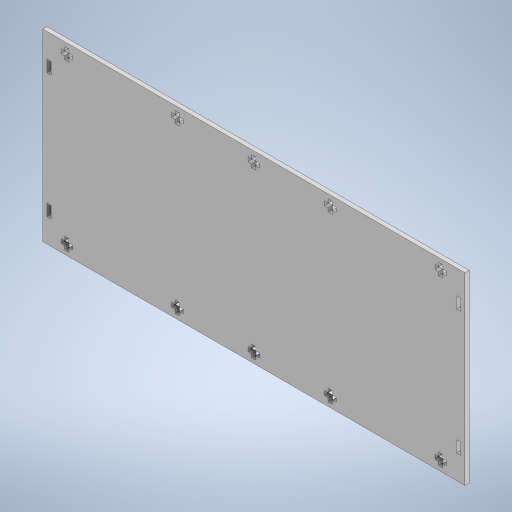
# Autodesk Inventor part: plate_expansion
Saved by Autodesk Inventor 2023 (Build 270158000, 158)
## iProperties
Created: 2023-05-04
Part Number: plate_expansion
Material: 一般
Document SubType Name: Modeling
Designer: 陳詩穎
Density: 1 g/cm^3
Appearance: 預設
Author: 陳詩穎
Autodesk Inventor part; units mm, degrees
ref_plane "YZ Plane" through (0, 0, 0) normal (1, 0, 0) x (0, 1, 0)
ref_plane "XZ Plane" through (0, 0, 0) normal (0, 1, 0) x (-1, 0, 0)
ref_plane "XY Plane" through (0, 0, 0) normal (0, 0, 1) x (1, 0, 0)
sketch "草圖1" plane through (0, 0, 0) normal (0, 0, 1) x (1, 0, 0)
  line L0 (-149, 65) -> (149, 65)
  line L1 (149, 65) -> (149, -65)
  line L2 (149, -65) -> (-149, -65)
  line L3 (-149, -65) -> (-149, 65)
  line L4 (0, -91) -> (0, 91) projected
  line L5 (-208.6, 0) -> (208.6, 0) projected
  point P0 (0, 0)
  dimension "d0" = 298
  dimension "d1" = 130
  constraints: 8 end point, 2 parallel, 1 horizontal, 1 perpendicular, 2 other
  measures "d0" distance of L0.start L0.end
  measures "d1" distance of L0.end L1.end
extrude "擠出1" add sketch "草圖1" along normal blind 3
sketch "草圖2" plane through (0, 0, 3) normal (0, 0, 1) x (1, 0, 0)
  line L0 (-1.45, 62) -> (1.45, 62)
  line L1 (1.45, 62) -> (1.45, 54)
  line L2 (1.45, 54) -> (-1.45, 54)
  line L3 (-1.45, 54) -> (-1.45, 62)
  line L4 (-4, 59.45) -> (4, 59.45)
  line L5 (4, 59.45) -> (4, 56.55)
  line L6 (4, 56.55) -> (-4, 56.55)
  line L7 (-4, 56.55) -> (-4, 59.45)
  line L8 (149, 65) -> (-149, 65) projected
  line L9 (1.45, 62) -> (-1.45, 54)
  line L10 (-1.45, 62) -> (1.45, 54)
  line L11 (4, 59.45) -> (-4, 56.55)
  line L12 (-4, 59.45) -> (4, 56.55)
  line L13 (-55.43, 62) -> (-52.53, 62)
  line L14 (-52.53, 62) -> (-52.53, 54)
  line L15 (-52.53, 54) -> (-55.43, 54)
  line L16 (-55.43, 54) -> (-55.43, 62)
  line L17 (-57.98, 59.45) -> (-49.98, 59.45)
  line L18 (-49.98, 59.45) -> (-49.98, 56.55)
  line L19 (-49.98, 56.55) -> (-57.98, 56.55)
  line L20 (-57.98, 56.55) -> (-57.98, 59.45)
  line L21 (-52.53, 62) -> (-55.43, 54)
  line L22 (-55.43, 62) -> (-52.53, 54)
  line L23 (-49.98, 59.45) -> (-57.98, 56.55)
  line L24 (-57.98, 59.45) -> (-49.98, 56.55)
  line L25 (-133.41, 62) -> (-130.51, 62)
  line L26 (-130.51, 62) -> (-130.51, 54)
  line L27 (-130.51, 54) -> (-133.41, 54)
  line L28 (-133.41, 54) -> (-133.41, 62)
  line L29 (-135.96, 56.55) -> (-135.96, 59.45)
  line L30 (-130.51, 62) -> (-133.41, 54)
  line L31 (-133.41, 62) -> (-130.51, 54)
  line L32 (-135.96, 59.45) -> (-127.96, 59.45)
  line L33 (-127.96, 56.55) -> (-135.96, 56.55)
  line L34 (-127.96, 59.45) -> (-135.96, 56.55)
  line L35 (-135.96, 59.45) -> (-127.96, 56.55)
  line L36 (-127.96, 59.45) -> (-127.96, 56.55)
  line L37 (-149, 65) -> (-149, -65) projected
  line L38 (-149, 0) -> (145, 0)
  line L39 (0, 65) -> (0, -65)
  line L40 (55.43, 62) -> (52.53, 62)
  line L41 (52.53, 62) -> (52.53, 54)
  line L42 (52.53, 54) -> (55.43, 54)
  line L43 (55.43, 54) -> (55.43, 62)
  line L44 (57.98, 56.55) -> (57.98, 59.45)
  line L45 (52.53, 62) -> (55.43, 54)
  line L46 (55.43, 62) -> (52.53, 54)
  line L47 (57.98, 59.45) -> (49.98, 59.45)
  line L48 (49.98, 56.55) -> (57.98, 56.55)
  line L49 (49.98, 59.45) -> (57.98, 56.55)
  line L50 (57.98, 59.45) -> (49.98, 56.55)
  line L51 (49.98, 59.45) -> (49.98, 56.55)
  line L52 (127.96, 59.45) -> (127.96, 56.55)
  line L53 (130.51, 62) -> (130.51, 54)
  line L54 (133.41, 54) -> (133.41, 62)
  line L55 (130.51, 62) -> (133.41, 54)
  line L56 (133.41, 62) -> (130.51, 54)
  line L57 (130.51, 54) -> (133.41, 54)
  line L58 (135.96, 59.45) -> (127.96, 59.45)
  line L59 (135.96, 59.45) -> (127.96, 56.55)
  line L60 (135.96, 56.55) -> (135.96, 59.45)
  line L61 (127.96, 56.55) -> (135.96, 56.55)
  line L62 (127.96, 59.45) -> (135.96, 56.55)
  line L63 (133.41, 62) -> (130.51, 62)
  line L64 (-1.45, -62) -> (1.45, -62)
  line L65 (1.45, -62) -> (1.45, -54)
  line L66 (1.45, -54) -> (-1.45, -54)
  line L67 (-1.45, -54) -> (-1.45, -62)
  line L68 (-4, -59.45) -> (4, -59.45)
  line L69 (4, -59.45) -> (4, -56.55)
  line L70 (4, -56.55) -> (-4, -56.55)
  line L71 (-4, -56.55) -> (-4, -59.45)
  line L72 (1.45, -62) -> (-1.45, -54)
  line L73 (-1.45, -62) -> (1.45, -54)
  line L74 (4, -59.45) -> (-4, -56.55)
  line L75 (-4, -59.45) -> (4, -56.55)
  line L76 (-55.43, -62) -> (-52.53, -62)
  line L77 (-52.53, -62) -> (-52.53, -54)
  line L78 (-52.53, -54) -> (-55.43, -54)
  line L79 (-55.43, -54) -> (-55.43, -62)
  line L80 (-57.98, -56.55) -> (-57.98, -59.45)
  line L81 (-52.53, -62) -> (-55.43, -54)
  line L82 (-55.43, -62) -> (-52.53, -54)
  line L83 (-57.98, -59.45) -> (-49.98, -59.45)
  line L84 (-49.98, -56.55) -> (-57.98, -56.55)
  line L85 (-49.98, -59.45) -> (-57.98, -56.55)
  line L86 (-57.98, -59.45) -> (-49.98, -56.55)
  line L87 (-49.98, -59.45) -> (-49.98, -56.55)
  line L88 (-127.96, -59.45) -> (-127.96, -56.55)
  line L89 (-130.51, -62) -> (-130.51, -54)
  line L90 (-133.41, -54) -> (-133.41, -62)
  line L91 (-130.51, -62) -> (-133.41, -54)
  line L92 (-133.41, -62) -> (-130.51, -54)
  line L93 (-130.51, -54) -> (-133.41, -54)
  line L94 (-135.96, -59.45) -> (-127.96, -59.45)
  line L95 (-135.96, -59.45) -> (-127.96, -56.55)
  line L96 (-135.96, -56.55) -> (-135.96, -59.45)
  line L97 (-127.96, -56.55) -> (-135.96, -56.55)
  line L98 (-127.96, -59.45) -> (-135.96, -56.55)
  line L99 (-133.41, -62) -> (-130.51, -62)
  line L100 (52.53, -62) -> (52.53, -54)
  line L101 (52.53, -62) -> (55.43, -54)
  line L102 (55.43, -62) -> (52.53, -54)
  line L103 (55.43, -62) -> (52.53, -62)
  line L104 (57.98, -56.55) -> (57.98, -59.45)
  line L105 (57.98, -59.45) -> (49.98, -59.45)
  line L106 (49.98, -56.55) -> (57.98, -56.55)
  line L107 (49.98, -59.45) -> (57.98, -56.55)
  line L108 (55.43, -54) -> (55.43, -62)
  line L109 (52.53, -54) -> (55.43, -54)
  line L110 (49.98, -59.45) -> (49.98, -56.55)
  line L111 (57.98, -59.45) -> (49.98, -56.55)
  line L112 (127.96, -59.45) -> (127.96, -56.55)
  line L113 (130.51, -54) -> (133.41, -54)
  line L114 (130.51, -62) -> (130.51, -54)
  line L115 (133.41, -62) -> (130.51, -62)
  line L116 (133.41, -54) -> (133.41, -62)
  line L117 (133.41, -62) -> (130.51, -54)
  line L118 (130.51, -62) -> (133.41, -54)
  line L119 (127.96, -56.55) -> (135.96, -56.55)
  line L120 (135.96, -59.45) -> (127.96, -59.45)
  line L121 (135.96, -59.45) -> (127.96, -56.55)
  line L122 (127.96, -59.45) -> (135.96, -56.55)
  line L123 (135.96, -56.55) -> (135.96, -59.45)
  line L124 (-146, 48) -> (-143.1, 48)
  line L125 (-143.1, 48) -> (-143.1, 40)
  line L126 (-143.1, 40) -> (-146, 40)
  line L127 (-146, 40) -> (-146, 48)
  line L128 (-146, -40) -> (-143.1, -40)
  line L129 (-143.1, -40) -> (-143.1, -48)
  line L130 (-143.1, -48) -> (-146, -48)
  line L131 (-146, -48) -> (-146, -40)
  line L132 (146, 48) -> (143.1, 48)
  line L133 (143.1, 48) -> (143.1, 40)
  line L134 (143.1, 40) -> (146, 40)
  line L135 (146, 40) -> (146, 48)
  line L136 (146, -40) -> (143.1, -40)
  line L137 (143.1, -40) -> (143.1, -48)
  line L138 (143.1, -48) -> (146, -48)
  line L139 (146, -48) -> (146, -40)
  point P0 (0, 0)
  point P1 (0, 58)
  point P2 (0, 58)
  point P3 (-53.98, 58)
  point P4 (-53.98, 58)
  point P5 (-53.98, 58)
  point P6 (0, 58)
  point P7 (-131.96, 58)
  point P8 (-131.96, 58)
  point P9 (-131.96, 58)
  point P10 (53.98, 58)
  point P11 (53.98, 58)
  point P12 (53.98, 58)
  point P13 (131.96, 58)
  point P14 (131.96, 58)
  point P15 (131.96, 58)
  point P16 (0, -58)
  point P17 (0, -58)
  point P18 (-53.98, -58)
  point P19 (-53.98, -58)
  point P20 (-53.98, -58)
  point P21 (0, -58)
  point P22 (-131.96, -58)
  point P23 (-131.96, -58)
  point P24 (-131.96, -58)
  point P25 (53.98, -58)
  point P26 (53.98, -58)
  point P27 (53.98, -58)
  point P28 (131.96, -58)
  point P29 (131.96, -58)
  point P30 (131.96, -58)
  point P31 (-133.41, -59.45)
  point P32 (-130.51, -59.45)
  point P33 (-130.51, -56.55)
  point P34 (-133.41, -56.55)
  point P35 (-55.43, -56.55)
  point P36 (-55.43, -59.45)
  point P37 (-52.53, -59.45)
  point P38 (-52.53, -56.55)
  point P39 (1.45, -56.55)
  point P40 (-1.45, -56.55)
  point P41 (-1.45, -59.45)
  point P42 (1.45, -59.45)
  point P43 (55.43, -59.45)
  point P44 (55.43, -56.55)
  point P45 (52.53, -56.55)
  point P46 (52.53, -59.45)
  point P47 (133.41, -56.55)
  point P48 (130.51, -56.55)
  point P49 (130.51, -59.45)
  point P50 (133.41, -59.45)
  point P51 (133.41, 59.45)
  point P52 (130.51, 59.45)
  point P53 (130.51, 56.55)
  point P54 (133.41, 56.55)
  point P55 (52.53, 56.55)
  point P56 (55.43, 56.55)
  point P57 (55.43, 59.45)
  point P58 (52.53, 59.45)
  point P59 (-1.45, 59.45)
  point P60 (-1.45, 56.55)
  point P61 (1.45, 56.55)
  point P62 (1.45, 59.45)
  point P63 (-52.53, 59.45)
  point P64 (-55.43, 59.45)
  point P65 (-55.43, 56.55)
  point P66 (-52.53, 56.55)
  point P67 (-130.51, 59.45)
  point P68 (-133.41, 59.45)
  point P69 (-133.41, 56.55)
  point P70 (-130.51, 56.55)
  dimension "d4" = 2.9
  dimension "d5" = 8
  dimension "d6" = 3
  dimension "d7" = 2.9
  dimension "d8" = 8
  dimension "d9" = 51.08
  dimension "d10" = 2.9
  dimension "d11" = 8
  dimension "d13" = 75.08
  dimension "d16" = 2.9
  dimension "d17" = 8
  dimension "d18" = 3
  dimension "d19" = 80
  constraints: 276 end point, 85 symmetric about line, 16 parallel, 14 midpoint, 14 perpendicular, 9 horizontal, 4 point on line, 2 horizontal alignment, 1 vertical, 1 vertical alignment, 2 other
  measures "d4" distance of L0.start L0.end
  measures "d5" distance of L0.end L1.end
  measures "d6" distance from line of L39.start L0
  measures "d7" distance of L13.start L13.end
  measures "d8" distance of L13.end L14.end
  measures "d9" distance between parallel lines of L14 L3
  measures "d10" distance of L28.end L26.start
  measures "d11" distance of L26.start L26.end
  measures "d13" distance between parallel lines of L26 L16
  measures "d16" distance of L124.start L124.end
  measures "d17" distance of L124.end L125.end
  measures "d18" distance between parallel lines of L37 L127
  measures "d19" distance between parallel lines of L128 L126
extrude "擠出2" cut sketch "草圖2" against normal blind 3 contours L10 L4 L3 | L0 L39 L4 L10 | L0 L9 L4 L39 | L4 L10 L12 L3 | L3 L12 L4 | L4 L39 L10 | L1 L4 L9 | L4 L9 L39 | L12 L11 L3 | L3 L11 L7 L12 | L39 L6 L9 | L12 L1 L6 L10 | L9 L4 L1 L11 | L9 L6 L3 L11 | L11 L1 L12 | L10 L6 L39 | L4 L11 L1 | L3 L6 L11 | L9 L3 L6 | L6 L39 L2 L9 | L10 L2 L39 L6 | L6 L1 L10 | L11 L5 L12 L1 | L12 L6 L1 | L22 L17 L16 | L13 L21 L17 L22 | L14 L17 L21 | L17 L22 L24 L16 | L16 L24 L17 | L17 L21 L22 | L17 L23 L14 | L14 L23 L21 L17 | L24 L23 L16 | L16 L23 L20 L24 | L22 L19 L21 | L24 L14 L19 L22 | L21 L19 L16 L23 | L23 L14 L24 | L23 L18 L24 L14 | L16 L19 L23 | L21 L16 L19 | L19 L22 L15 L21 | L19 L14 L22 | L24 L19 L14 | L31 L32 L28 | L25 L30 L32 L31 | L26 L32 L30 | L32 L31 L35 L28 | L28 L35 L32 | L32 L30 L31 | L32 L34 L26 | L26 L34 L30 L32 | L35 L34 L28 | L28 L34 L29 L35 | L31 L33 L30 | L35 L26 L33 L31 | L30 L33 L28 L34 | L34 L26 L35 | L34 L36 L35 L26 | L28 L33 L34 | L33 L31 L27 L30 | L30 L28 L33 | L33 L26 L31 | L35 L33 L26 | L66 L73 L70 L39 | L39 L70 L72 L66 | L70 L73 L39 | L39 L72 L70 | L65 L70 L73 | L72 L70 L67 | L72 L68 L39 | L74 L65 L68 L72 | L74 L67 L70 L72 | L39 L68 L73 | L75 L65 L74 | L75 L67 L74 | L73 L68 L67 L75 | L73 L70 L65 L75 | L70 L75 L65 | L67 L74 L70 | L68 L72 L64 L39 | L39 L64 L73 L68 | L68 L65 L72 | L73 L67 L68 | L74 L68 L65 | L65 L75 L69 L74 | L67 L75 L71 L74 | L67 L68 L75 | L46 L47 L45 L40 | L43 L47 L46 | L45 L47 L41 | L47 L50 L43 | L43 L50 L46 L47 | L46 L45 L47 | L47 L45 L49 L41 | L41 L49 L47 | L50 L44 L49 L43 | L43 L49 L50 | L49 L43 L48 L45 | L45 L48 L46 | L50 L41 L49 | L46 L48 L41 L50 | L41 L50 L51 L49 | L49 L48 L43 | L48 L43 L45 | L45 L42 L46 L48 | L46 L41 L48 | L41 L48 L50 | L62 L53 L59 L52 | L58 L53 L62 | L59 L53 L61 | L58 L55 L62 L53 | L53 L55 L58 | L62 L59 L53 | L59 L56 L61 L53 | L61 L56 L53 | L63 L56 L58 L55 | L58 L56 L55 | L62 L54 L61 L55 | L55 L61 L56 | L56 L58 L54 L59 | L59 L54 L62 | L56 L61 L55 L57 | L54 L58 L56 | L61 L54 L55 | L59 L60 L62 L54 | L54 L58 L59 | L62 L61 L54 | L82 L83 L81 L76 | L79 L83 L82 | L81 L83 L77 | L83 L86 L79 | L79 L86 L82 L83 | L82 L81 L83 | L83 L81 L85 L77 | L77 L85 L83 | L86 L80 L85 L79 | L79 L85 L86 | L85 L79 L84 L81 | L81 L84 L82 | L86 L77 L85 | L82 L84 L77 L86 | L77 L86 L87 L85 | L85 L84 L79 | L84 L79 L81 | L81 L78 L82 L84 | L82 L77 L84 | L77 L84 L86 | L98 L89 L95 L88 | L94 L89 L98 | L95 L89 L97 | L94 L91 L98 L89 | L89 L91 L94 | L98 L95 L89 | L95 L92 L97 L89 | L97 L92 L89 | L99 L92 L94 L91 | L94 L92 L91 | L98 L90 L97 L91 | L91 L97 L92 | L92 L94 L90 L95 | L95 L90 L98 | L92 L97 L91 L93 | L90 L94 L92 | L97 L90 L91 | L95 L96 L98 L90 | L90 L94 L95 | L98 L97 L90 | L100 L105 L101 | L101 L105 L102 L103 | L105 L107 L100 | L100 L107 L101 L105 | L101 L102 L105 | L102 L105 L108 | L107 L110 L111 L100 | L100 L111 L107 | L102 L106 L101 | L111 L108 L105 L102 | L111 L100 L106 L102 | L101 L106 L108 L107 | L107 L108 L111 | L108 L111 L105 | L111 L106 L100 | L106 L102 L109 L101 | L101 L108 L106 | L106 L100 L102 | L108 L106 L107 | L107 L104 L111 L108 | L122 L114 L120 | L112 L121 L114 L122 | L119 L114 L121 | L120 L118 L114 | L114 L122 L118 L120 | L114 L121 L122 | L119 L117 L121 L114 | L114 L117 L119 | L118 L120 L117 L115 | L118 L117 L120 | L121 L116 L120 L117 | L117 L119 L118 | L122 L116 L121 | L118 L119 L116 L122 | L113 L118 L119 L117 | L117 L120 L116 | L118 L116 L119 | L121 L120 L116 | L116 L122 L123 L121 | L116 L119 L122 | L124 L125 L126 L127 | L128 L129 L130 L131 | L135 L134 L133 L132 | L139 L138 L137 L136
